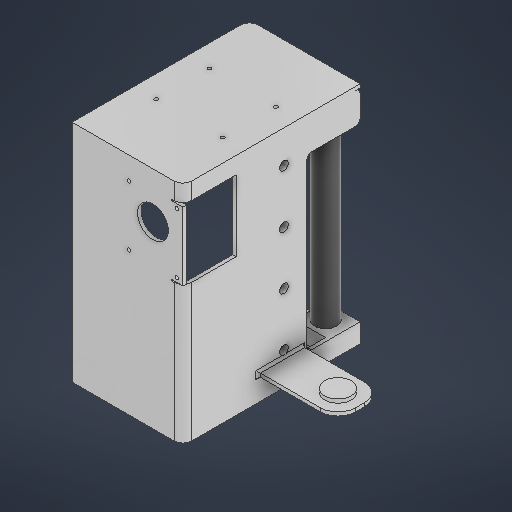
# Autodesk Inventor part: SACMI DPA TILES GRIP BASE
Saved by Autodesk Inventor 2025 (Build 290162000, 162)
## iProperties
Created: 2024-05-26
Part Number: SACMI DPA TILES GRIP BASE
Material: Generic
Document SubType Name: Modeling
Designer: zulet
Density: 1 g/cm^3
Appearance: Default
Author: zulet
Autodesk Inventor part; units mm, degrees
ref_plane "YZ Plane" through (0, 0, 0) normal (1, 0, 0) x (0, 1, 0)
ref_plane "XZ Plane" through (0, 0, 0) normal (0, 1, 0) x (-1, 0, 0)
sketch "Sketch1" plane through (0, 0, 0) normal (0, 1, 0) x (-1, 0, 0)
  line L0 (-105, 200) -> (125, 200)
  line L1 (125, 200) -> (125, -180)
  line L2 (105, -200) -> (-125, -200)
  line L3 (-125, -200) -> (-125, 180)
  line L4 (-125, 200) -> (125, -200) construction
  line L5 (125, 200) -> (-125, -200) construction
  arc A0 (105, -200) -> (125, -180) centre (105, -180) ccw
  arc A1 (-105, 200) -> (-125, 180) centre (-105, 180) ccw
  line L6 (-117, -192) -> (105, -192) construction
  arc A2 (105, -192) -> (117, -180) centre (105, -180) ccw construction
  line L7 (117, -180) -> (117, 192) construction
  line L8 (117, 192) -> (-105, 192)
  arc A3 (-105, 192) -> (-117, 180) centre (-105, 180) ccw
  line L9 (-117, 180) -> (-117, -192)
  line L10 (-117, -192) -> (-117, -200)
  line L11 (117, 192) -> (125, 192)
  point P0 (0, 0)
  dimension "d0" = 250
  dimension "d1" = 400
  dimension "d2" = 20
  dimension "d3" = 8
  constraints: 24 end point, 8 point on circle, 6 point on line, 4 centre point, 4 parallel, 4 perpendicular, 4 tangent, 2 midpoint, 1 equal radius, 1 horizontal, 5 other
  measures "d0" distance of L4.end L2.end
  measures "d1" distance of L0.end L4.end
  measures "d2" radius of A0
  measures "d3" distance between parallel lines of L2 L6
extrude "Extrusion1" add sketch "Sketch1" along normal blind 8 contours L1 A0 L2 L10 L9 A3 L8 L11
extrude "Extrusion2" add sketch "Sketch1" along normal blind 500 contours L0 L1 L11 L8 A3 L9 L10 L2 L3 A1
sketch "Sketch2" plane through (0, 8, 0) normal (0, 1, 0) x (1, 0, 0)
  line L0 (117, 200) -> (-105, 200) projected
  line L1 (117, 200) -> (47, 200)
  line L2 (47, 200) -> (47, 130)
  line L3 (47, 130) -> (117, 130)
  line L4 (117, 130) -> (117, 200)
  point P0 (0, 0)
  dimension "d8" = 70
  dimension "d9" = 70
  constraints: 8 end point, 2 parallel, 1 horizontal, 1 perpendicular
  measures "d8" distance of L3.end L2.end
  measures "d9" distance of L2.end L1.end
extrude "Extrusion3" add sketch "Sketch2" along normal blind 35
sketch "Sketch3" plane through (125, 0, 180) normal (1, 0, 0) x (0, 0, -1)
  line L0 (380, 43) -> (310, 43) projected
  line L1 (380, 43) -> (260, 43)
  line L2 (260, 43) -> (260, 430)
  line L3 (260, 430) -> (380, 430)
  line L4 (380, 430) -> (380, 43)
  line L5 (310, 43) -> (310, 8) projected
  line L6 (0, 500) -> (380, 500) construction
  point P0 (180, 0)
  dimension "d12" = 70
  dimension "d13" = 120
  constraints: 8 end point, 2 parallel, 1 horizontal, 1 perpendicular
  measures "d12" distance between parallel lines of L6 L3
  measures "d13" distance between parallel lines of L4 L2
extrude "Extrusion4" cut sketch "Sketch3" against normal through all
fillet "Fillet1" radius 10 4 edges at (121, 430, -200) (121, 430, -80) (121, 500, -200) (121, 43, -80)
sketch "Sketch4" plane through (0, 43, 0) normal (0, 1, 0) x (1, 0, 0)
  line L0 (47, 130) -> (47, 200) construction
  line L1 (47, 200) -> (-105, 200) projected
  arc A0 (-105, 200) -> (-125, 180) centre (-105, 180) ccw projected
  line L2 (-125, 180) -> (-125, -192) projected
  line L3 (-125, -192) -> (105, -192) projected
  arc A1 (105, -192) -> (117, -180) centre (105, -180) ccw projected
  line L4 (117, -180) -> (117, 130) projected
  line L5 (117, 130) -> (47, 130) construction
  line L6 (125, 200) -> (117, 200) construction
  line L7 (47, 130) -> (117, 130) construction
  line L8 (117, 130) -> (117, 200) construction
  line L9 (117, 200) -> (47, 200) construction
  line L10 (47, 200) -> (47, 130) construction
  line L11 (117, 130) -> (47, 200) construction
  line L12 (47, 130) -> (117, 200) construction
  circle A2 centre (82, 165) radius 25
  point P0 (0, 0)
  dimension "d17" = 50
  constraints: 12 end point, 2 parallel, 2 perpendicular, 1 centre point, 1 horizontal, 1 midpoint
  measures "d17" diameter of A2
extrude "Extrusion5" add sketch "Sketch4" along normal up to surface (387 mm away)
sketch "Sketch5" plane through (82, 430, -165) normal (0, 1, 0) x (1, 0, 0)
  line L0 (35, 25) -> (35, -75) projected
  line L1 (-35, -35) -> (35, -35) projected
  line L2 (-35, 35) -> (-35, -35) projected
  line L3 (-35, 35) -> (43, 35) projected
  line L4 (35, 25) -> (35, 35) projected
  point P0 (-82, -165)
extrude "Extrusion6" add sketch "Sketch5" along normal up to surface (70 mm away) separate body
sketch "Sketch7" plane through (117, 8, 180) normal (-1, 0, 0) x (0, 0, 1)
  line L0 (-370, 492) -> (0, 492) projected
  line L1 (-208, 492) -> (-208, 0) construction
  circle A0 centre (-208, 426) radius 10
  line L2 (12, 0) -> (12, 492) projected
  line L3 (0, 0) -> (-310, 0) projected
  circle A1 centre (-208, 306) radius 10
  circle A2 centre (-208, 186) radius 10
  circle A3 centre (-208, 66) radius 10
  line L4 (20, -8) -> (20, 492) projected
  line L5 (20, 462) -> (-100, 462)
  line L6 (-100, 462) -> (-100, 302)
  line L7 (-100, 302) -> (20, 302)
  line L8 (20, 302) -> (20, 462)
  point P0 (-180, -8)
  point P1 (20, 382)
  point P2 (20, 302)
  point P3 (-100, 382)
  dimension "d23" = 20
  dimension "d27" = 220
  dimension "d32" = 120
  dimension "d37" = 66
  dimension "d38" = 66
  dimension "d39" = 160
  dimension "d40" = 120
  dimension "d62" = 110
  constraints: 10 end point, 4 centre point, 4 point on line, 2 midpoint, 2 parallel, 2 vertical, 1 horizontal, 1 perpendicular, 6 other
  measures "d23" diameter of A0
  measures "d27" distance between parallel lines of L2 L1
  measures "d32" distance of A0.centre A1.centre
  measures "d37" distance from line of L0 A0.centre
  measures "d38" distance from line of L3 A3.centre
  measures "d39" distance of L5.end L6.end
  measures "d40" distance of L5.start L5.end
  measures "d62" distance from line of L0 point (-100, 382)
extrude "Extrusion7" cut sketch "Sketch7" against normal through all contours A0 | A1 | A2 | A3 bodies 1
extrude "Extrusion8" cut sketch "Sketch7" along normal mid plane 35 contours L7 L6 L5 L2 | L2 L5 L4 L7 bodies 1
sketch "Sketch8" plane through (99.5, 8, 180) normal (1, 0, 0) x (0, 0, -1)
  line L0 (-20, 302) -> (-20, 462) projected
  line L1 (-12, 462) -> (-12, 302) projected
  line L2 (-20, 459) -> (-12, 459)
  line L3 (-12, 459) -> (-12, 305)
  line L4 (-12, 305) -> (-20, 305)
  line L5 (-20, 305) -> (-20, 459)
  line L6 (0, 462) -> (-20, 462) projected
  line L7 (-20, 302) -> (0, 302) projected
  point P0 (180, -8)
  point P1 (-20, 305)
  point P2 (-12, 459)
  dimension "d43" = 3
  dimension "d44" = 3
  constraints: 8 end point, 2 parallel, 2 point on line, 1 horizontal, 1 perpendicular
  measures "d43" distance between parallel lines of L6 L2
  measures "d44" distance between parallel lines of L7 L4
extrude "Extrusion9" add sketch "Sketch8" along normal up to surface (25.5 mm away) contours L0 L2 L1 L4 bodies 1
sketch "Sketch9" plane through (-125, 0, 200) normal (0, 0, 1) x (1, 0, 0)
  circle A0 centre (182.5, 390) radius 35 construction
  line L0 (250, 313) -> (250, 467) projected
  line L1 (236.5, 322.5) -> (128.5, 322.5) construction
  line L2 (128.5, 322.5) -> (128.5, 457.5) construction
  line L3 (128.5, 457.5) -> (236.5, 457.5) construction
  line L4 (236.5, 457.5) -> (236.5, 322.5) construction
  line L5 (236.5, 322.5) -> (128.5, 457.5) construction
  line L6 (128.5, 322.5) -> (236.5, 457.5) construction
  line L7 (182.5, 390) -> (250, 390) construction
  line L8 (182.5, 390) -> (182.5, 404.5) construction
  circle A1 centre (182.5, 404.5) radius 35
  point P0 (125, 0)
  dimension "d47" = 67.5
  dimension "d48" = 108
  dimension "d49" = 135
  dimension "d50" = 70
  dimension "d60" = 14.5
  dimension "d61" = 70
  constraints: 16 end point, 5 coincident, 3 midpoint, 2 centre point, 2 horizontal, 2 parallel, 1 perpendicular, 1 vertical
  measures "d47" distance from line of L0 L7.start
  measures "d48" distance of L2.end L3.end
  measures "d49" distance of L1.end L2.end
  measures "d50" diameter of A0
  measures "d60" distance of L7.start L8.end
  measures "d61" diameter of A1
hole "Hole1" at (3.5, 457.5, 200) at (111.5, 457.5, 200) at (111.5, 322.5, 200) at (3.5, 322.5, 200) direction (0, 0, -1) diameter 8 depth 15 bodies 1
extrude "Extrusion10" cut sketch "Sketch9" against normal blind 10 bodies 1
sketch "Sketch10" plane through (117, 8, -130) normal (-1, 0, 0) x (0, 0, 1)
  line L0 (-60, 492) -> (310, 492) projected
  line L1 (310, 0) -> (0, 0) projected
  line L2 (67, 492) -> (137, 492)
  line L3 (137, 492) -> (137, 0)
  line L4 (137, 0) -> (67, 0)
  line L5 (67, 0) -> (67, 492)
  circle A0 centre (102, 426) radius 10 projected
  circle A1 centre (102, 306) radius 10 projected
  circle A2 centre (102, 186) radius 10 projected
  circle A3 centre (102, 66) radius 10 projected
  point P0 (130, -8)
  point P1 (67, 0)
  dimension "d63" = 35
  dimension "d64" = 35
  constraints: 8 end point, 2 parallel, 2 point on line, 1 horizontal, 1 perpendicular
  measures "d63" distance from line of L5 A0.centre
  measures "d64" distance from line of L3 A0.centre
extrude "Extrusion11" add sketch "Sketch10" along normal blind 30 bodies 1
sketch "Sketch11" plane through (0, 500, 0) normal (0, 1, 0) x (1, 0, 0)
  line L0 (-125, 180) -> (-125, -200) projected
  arc A0 (-105, 200) -> (-125, 180) centre (-105, 180) ccw projected
  line L1 (125, 200) -> (-105, 200) projected
  line L2 (125, -180) -> (125, 200) projected
  arc A1 (105, -200) -> (125, -180) centre (105, -180) ccw projected
  line L3 (-125, -200) -> (105, -200) projected
  point P0 (0, 0)
extrude "Extrusion12" add sketch "Sketch11" along normal blind 8 bodies 1
sketch "Sketch12" plane through (0, 508, 0) normal (0, 1, 0) x (1, 0, 0)
  line L0 (-75, 60) -> (75, 60) construction
  line L1 (75, 60) -> (75, -60) construction
  line L2 (75, -60) -> (-75, -60) construction
  line L3 (-75, -60) -> (-75, 60) construction
  line L4 (-75, 60) -> (75, -60) construction
  line L5 (75, 60) -> (-75, -60) construction
  point P0 (0, 0)
  dimension "d69" = 150
  dimension "d70" = 120
  constraints: 12 end point, 4 coincident, 2 midpoint, 2 parallel, 1 horizontal, 1 perpendicular
  measures "d69" distance of L1.end L2.end
  measures "d70" distance of L0.end L1.end
hole "Hole2" at (75, 508, -60) at (75, 508, 60) at (-75, 508, 60) at (-75, 508, -60) direction (0, -1, 0) diameter 8 depth 8 tip angle 118 bodies 1
ref_plane "Work Plane1" through (0, 60, 0) normal (0, -1, 0) x (1, 0, 0)
sketch "Sketch13" plane through (0, 60, 0) normal (0, -1, 0) x (1, 0, 0)
  line L0 (125, 180) -> (125, -200) projected
  line L1 (125, 30) -> (305, 30)
  line L2 (305, 30) -> (305, -70)
  line L3 (305, -70) -> (125, -70)
  line L4 (125, -70) -> (125, 30)
  line L5 (47, -200) -> (125, -200) projected
  line L6 (305, 30) -> (205, -70) construction
  line L7 (305, -70) -> (205, 30) construction
  line L8 (205, 30) -> (205, -70) construction
  circle A0 centre (255, -20) radius 30
  point P0 (0, 0)
  dimension "d79" = 180
  dimension "d80" = 100
  dimension "d81" = 130
  dimension "d82" = 100
  dimension "d83" = 60
  constraints: 14 end point, 3 point on line, 2 parallel, 2 perpendicular, 1 centre point, 1 horizontal, 1 midpoint
  measures "d79" distance of L2.end L3.end
  measures "d80" distance of L1.end L2.end
  measures "d81" distance between parallel lines of L5 L3
  measures "d82" distance between parallel lines of L2 L8
  measures "d83" diameter of A0
extrude "Extrusion13" add sketch "Sketch13" along normal blind 8 contours L1 L2 L3 L0 | A0 bodies 1
extrude "Extrusion14" add sketch "Sketch13" against normal blind 8 contours A0 bodies 1
fillet "Fillet2" radius 40 2 edges at (305, 56, 30) (305, 56, -70)
fillet "Fillet3" radius 5 4 edges at (125, 60, -20) (125, 52, -20) (125, 56, -70) (125, 56, 30)
equation "\"d4\" = d3"
equation "\"d37\" = d38"
equation "\"d82\" = d80"
body "Solid1"
body "Solid2"
